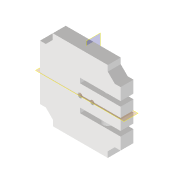
# Autodesk Inventor part: 20_Cube_Insert_2D_Galvo_Fiberlaunch_v3
Saved by Autodesk Inventor 2022 (Build 260153000, 153)
## iProperties
Created: 2019-07-01
Part Number: 20_Cube_Insert_2D_Galvo_Fiberlaunch_v3
Material: Generic
Document SubType Name: Modeling
Designer: diederichbenedict
Density: 1 g/cm^3
Appearance: Default
Author: diederichbenedict
Autodesk Inventor part; units mm, degrees
ref_plane "YZ Plane" through (0, 0, 0) normal (1, 0, 0) x (0, 1, 0)
ref_plane "XZ Plane" through (0, 0, 0) normal (0, 1, 0) x (-1, 0, 0)
ref_plane "Work Plane1" through (-56.3599, 0, 22) normal (0, 0, -1) x (-1, 0, 0)
sketch "Sketch1" plane through (-56.3599, 0, 22) normal (0, 0, -1) x (-1, 0, 0)
  line L0 (-4.0299, -0.3538) -> (-2.2322, 1.4439) construction
  arc A0 (-1.4439, 2.2322) -> (-2.2322, 1.4439) centre (-0.9299, 0.9299) ccw construction
  line L1 (-1.4439, 2.2322) -> (0.3538, 4.0299) construction
  line L2 (-37.8299, 42.8299) -> (-37.8299, 37.8299) construction
  line L3 (-37.8299, 37.8299) -> (-42.9208, 37.8299) construction
  line L4 (-37.8299, 42.2137) -> (-37.8299, 45.8299) construction
  line L5 (-37.8299, 45.8299) -> (-4.0299, 45.8299) construction
  line L6 (-4.0299, 45.8299) -> (-4.0299, 42.2137) construction
  line L7 (-4.0299, 4.0299) -> (0.3538, 4.0299) projected
  circle A1 centre (-20.9299, 20.9299) radius 17.5 projected
  line L8 (-20.9299, 58.9723) -> (17.1124, 20.9299) construction
  line L9 (17.1124, 20.9299) -> (-20.9299, -17.1124) construction
  line L10 (-20.9299, -17.1124) -> (-58.9723, 20.9299) construction
  line L11 (-58.9723, 20.9299) -> (-20.9299, 58.9723) construction
  line L12 (-20.9299, 58.9723) -> (-20.9299, -17.1124) construction
  line L13 (17.1124, 20.9299) -> (-58.9723, 20.9299) construction
  line L14 (-20.9299, 58.9723) -> (32.8701, 58.9723) construction
  line L15 (-43.4299, 43.4299) -> (1.5701, 43.4299) construction
  line L16 (1.5701, 43.4299) -> (1.5701, -1.5701) construction
  line L17 (1.5701, -1.5701) -> (-43.4299, -1.5701) construction
  line L18 (-43.4299, -1.5701) -> (-43.4299, 43.4299) construction
  line L19 (-43.4299, 43.4299) -> (1.5701, -1.5701) construction
  line L20 (1.5701, 43.4299) -> (-43.4299, -1.5701) construction
  line L21 (-43.4299, 5.3876) -> (-43.4299, 36.4723)
  line L22 (-43.4299, 36.4723) -> (-36.4723, 43.4299)
  line L23 (-36.4723, 43.4299) -> (-5.3876, 43.4299)
  line L24 (-5.3876, 43.4299) -> (1.5701, 36.4723)
  line L25 (1.5701, 36.4723) -> (1.5701, 5.3876)
  line L26 (1.5701, 5.3876) -> (-5.3876, -1.5701)
  line L27 (-5.3876, -1.5701) -> (-36.4723, -1.5701)
  line L28 (-36.4723, -1.5701) -> (-43.4299, 5.3876)
  line L29 (-4.0299, 42.2137) -> (-37.8299, 42.2137) projected
  line L30 (-4.0299, -0.3538) -> (-4.0299, 4.0299) projected
  circle A2 centre (-20.9299, 20.9299) radius 1.5
  line L31 (-10.9299, 10.9299) -> (-30.9299, 10.9299) construction
  line L32 (-30.9299, 10.9299) -> (-30.9299, 30.9299) construction
  line L33 (-30.9299, 30.9299) -> (-10.9299, 30.9299) construction
  line L34 (-10.9299, 30.9299) -> (-10.9299, 10.9299) construction
  line L35 (-10.9299, 10.9299) -> (-30.9299, 30.9299) construction
  line L36 (-30.9299, 10.9299) -> (-10.9299, 30.9299) construction
  circle A3 centre (-30.9299, 30.9299) radius 1.4
  circle A4 centre (-30.9299, 10.9299) radius 1.4
  circle A5 centre (-10.9299, 10.9299) radius 1.4
  line L37 (-45.8299, 37.8299) -> (-42.0723, 37.8299) construction
  line L38 (-42.1723, 37.7299) -> (-45.8299, 37.7299)
  line L39 (-45.8299, 37.7299) -> (-45.8299, 4.1299)
  line L40 (-45.8299, 4.1299) -> (-42.1723, 4.1299)
  line L41 (-42.1723, 4.1299) -> (-42.1723, 37.7299)
  line L42 (-45.8299, 4.0299) -> (-42.0723, 4.0299) construction
  line L43 (-45.8299, 37.8299) -> (-42.0723, 37.8299) projected
  line L44 (-37.7299, 45.8299) -> (-4.1299, 45.8299)
  line L45 (-4.1299, 45.8299) -> (-4.1299, 42.1723)
  line L46 (-4.1299, 42.1723) -> (-37.7299, 42.1723)
  line L47 (-37.7299, 42.1723) -> (-37.7299, 45.8299)
  line L48 (0.4701, 37.8299) -> (0.4701, 4.0299) construction
  line L49 (0.4701, 4.0299) -> (3.9701, 4.0299) construction
  line L50 (3.9701, 37.8299) -> (3.9701, 4.0299) construction
  line L51 (0.4701, 37.8299) -> (3.9701, 37.8299) construction
  line L52 (-45.8299, -3.9701) -> (-4.0299, -3.9701) construction
  line L53 (0.3124, 37.7299) -> (3.9701, 37.7299)
  line L54 (3.9701, 37.7299) -> (3.9701, 4.1299)
  line L55 (3.9701, 4.1299) -> (0.3124, 4.1299)
  line L56 (0.3124, 4.1299) -> (0.3124, 37.7299)
  line L57 (-4.1713, -0.3538) -> (-37.7299, -0.3538)
  line L58 (-37.7299, -0.3538) -> (-37.7299, -3.9701)
  line L59 (-37.7299, -3.9701) -> (-4.1713, -3.9701)
  line L60 (-4.1713, -3.9701) -> (-4.1713, -0.3538)
  point P0 (-37.8299, 4.0299)
  dimension "d18" = 53.8
  dimension "d19" = 45
  dimension "d20" = 53.8
  dimension "d21" = 45
  dimension "d22" = 45
  dimension "d30" = 20
  dimension "d31" = 20
  dimension "d32" = 2.8
  dimension "d33" = 2.8
  dimension "d34" = 2.8
  dimension "d35" = 3
  dimension "d36" = 0.1
  dimension "d37" = 0.1
  dimension "d38" = 0.1
  dimension "d39" = 0.1
  constraints: 86 end point, 21 point on line, 14 parallel, 8 perpendicular, 7 horizontal, 7 midpoint, 4 centre point, 4 coincident, 1 equal length
  measures "d18" distance of L8.start L8.end
  measures "d19" angle of L8 L14
  measures "d20" distance of L8.end L9.end
  measures "d21" distance of L16.end L17.end
  measures "d22" distance of L15.end L16.end
  measures "d30" distance of L32.end L33.end
  measures "d31" distance of L31.end L32.end
  measures "d32" diameter of A3
  measures "d33" diameter of A4
  measures "d34" diameter of A5
  measures "d35" diameter of A2
  measures "d36" distance between parallel lines of L38 L43
  measures "d37" distance between parallel lines of L40 L42
  measures "d38" distance between parallel lines of L45 L6
  measures "d39" distance between parallel lines of L4 L47
extrude "Extrusion1" add sketch "Sketch1" along normal blind 8 contours L30 L26 L57 L28 L41 L22 L46 L24 L56 L7 | L7 L26 L30 | L56 L24 L25 L26 | L26 L25 L24 L53 L54 L55 | L60 L59 L58 L57 L28 L27 L26 | L26 L27 L28 L57 | L46 L22 L29 L24 | L24 L29 L45 | L40 L39 L38 L22 L21 L28 | L28 L21 L22 L41 | L29 L22 L23 L24 | L24 L23 L22 L29 L47 L44 L45 | L47 L29 L22 | A1 | A2 | A3 | A4 | A5
sketch "Skizze4" plane through (-56.3599, 0, 14) normal (0, 0, -1) x (-1, 0, 0)
  line L0 (-37.7299, 42.1723) -> (-42.1723, 37.7299) projected
  line L1 (-42.1723, 37.7299) -> (-45.8299, 37.7299) projected
  line L2 (-45.8299, 37.7299) -> (-45.8299, 4.1299) construction
  line L3 (-45.8299, 4.1299) -> (-42.1723, 4.1299) projected
  line L4 (-42.1723, 4.1299) -> (-37.6885, -0.3538) projected
  line L5 (-37.6885, -0.3538) -> (-37.7299, -0.3538) projected
  line L6 (-37.7299, -0.3538) -> (-37.7299, -3.9701) projected
  line L7 (-37.7299, -3.9701) -> (-4.1713, -3.9701) construction
  line L8 (-4.1713, -3.9701) -> (-4.1713, -0.3538) projected
  line L9 (-4.1713, -0.3538) -> (0.3124, 4.1299) projected
  line L10 (0.3124, 4.1299) -> (3.9701, 4.1299) projected
  line L11 (3.9701, 4.1299) -> (3.9701, 37.7299) construction
  line L12 (3.9701, 37.7299) -> (0.3124, 37.7299) projected
  line L13 (0.3124, 37.7299) -> (-4.1299, 42.1723) projected
  line L14 (-4.1299, 42.1723) -> (-4.1299, 45.8299) projected
  line L15 (-4.1299, 45.8299) -> (-37.7299, 45.8299) construction
  line L16 (-37.7299, 45.8299) -> (-37.7299, 42.1723) projected
  line L17 (-37.9299, 46.0299) -> (-3.9299, 46.0299) construction
  line L18 (-3.9299, 46.0299) -> (-3.9299, 42.2551)
  line L19 (-3.9299, 42.2551) -> (0.3953, 37.9299)
  line L20 (0.3953, 37.9299) -> (4.1701, 37.9299)
  line L21 (4.1701, 37.9299) -> (4.1701, 3.9299) construction
  line L22 (4.1701, 3.9299) -> (0.3953, 3.9299)
  line L23 (0.3953, 3.9299) -> (-3.9713, -0.4367)
  line L24 (-3.9713, -0.4367) -> (-3.9713, -4.1701)
  line L25 (-3.9713, -4.1701) -> (-37.9299, -4.1701) construction
  line L26 (-37.9299, -4.1701) -> (-37.9299, -0.3953)
  line L27 (-37.9299, -0.3953) -> (-42.2551, 3.9299)
  line L28 (-42.2551, 3.9299) -> (-46.0299, 3.9299)
  line L29 (-46.0299, 3.9299) -> (-46.0299, 37.9299) construction
  line L30 (-46.0299, 37.9299) -> (-42.2551, 37.9299)
  line L31 (-42.2551, 37.9299) -> (-37.9299, 42.2551)
  line L32 (-37.9299, 42.2551) -> (-37.9299, 46.0299)
  line L33 (-45.8299, 37.7299) -> (-45.8299, 37.9299)
  line L34 (-4.1299, 45.8299) -> (-37.7299, 45.8299) projected
  line L35 (-37.7299, 45.8299) -> (-37.9299, 45.8299)
  line L36 (-4.1299, 45.8299) -> (-3.9299, 45.8299)
  line L37 (3.9701, 37.7299) -> (3.9701, 37.9299)
  line L38 (3.9701, 4.1299) -> (3.9701, 37.7299) projected
  line L39 (3.9701, 4.1299) -> (3.9701, 3.9299)
  line L40 (-4.1713, -3.9701) -> (-3.9713, -3.9701)
  line L41 (-37.7299, -3.9701) -> (-37.9299, -3.9701)
  line L42 (-45.8299, 4.1299) -> (-45.8299, 3.9299)
  point P0 (-56.3599, 0)
  dimension "d40" = 0.2
  constraints: 48 end point, 12 point on line, 4 perpendicular, 15 other
  measures "d40" distance between parallel lines of L15 L17
extrude "IM_offset" add sketch "Skizze4" against normal up to surface (8 mm away)
ref_plane "Arbeitsebene5" through (-35.4299, 3.9299, 22) normal (-1, 0, 0) x (0, 0, 1)
ref_plane "Arbeitsebene6" through (-18.4299, 20.9299, 22) normal (0, 1, 0) x (-1, 0, 0)
sketch "Skizze31" plane through (-56.3599, 0, 22) normal (0, 0, 1) x (1, 0, 0)
  line L0 (25.9049, 44.8899) -> (15.7949, 44.8899) projected
  spline S0 degree 3 poles (21.2744, 21.9194) (21.3357, 21.9462) (21.3936, 21.9718) (21.5033, 22.0154) (21.5491, 22.0289) (21.5827, 22.0289) (21.5892, 22.0276) (21.5935, 22.0247) knots 0.300335 0.300335 0.300335 0.300335 0.323424 0.323424 0.35266 0.35266 0.362351 0.362351 0.362351 0.362351 projected
  line L1 (21.2744, 21.9194) -> (21.2744, 26.3899) projected
  line L2 (20.4254, 21.9194) -> (20.4254, 26.3899) projected
  line L3 (21.9714, 15.3899) -> (21.1087, 15.3899) projected
  line L4 (20.5911, 15.3899) -> (19.7285, 15.3899) projected
  line L5 (20.5999, 15.3899) -> (21.0999, 15.3899) projected
  line L6 (28.5999, 22.8289) -> (28.5999, 24.3299) projected
  line L7 (28.5999, 24.3299) -> (28.0999, 24.3299) projected
  line L8 (28.0999, 24.3299) -> (28.0999, 22.8289) projected
  line L9 (28.0999, 22.8289) -> (27.7114, 24.2788) projected
  line L10 (27.7114, 24.2788) -> (27.2285, 24.1494) projected
  line L11 (27.2285, 24.1494) -> (28.0911, 20.9299) projected
  line L12 (28.0911, 20.9299) -> (27.2285, 17.7105) projected
  line L13 (27.2285, 17.7105) -> (27.7114, 17.5811) projected
  line L14 (27.7114, 17.5811) -> (28.0999, 19.031) projected
  line L15 (28.0999, 19.031) -> (28.0999, 17.5299) projected
  line L16 (28.0999, 17.5299) -> (28.5999, 17.5299) projected
  line L17 (28.5999, 17.5299) -> (28.5999, 19.031) projected
  line L18 (28.5999, 19.031) -> (28.9884, 17.5811) projected
  line L19 (28.9884, 17.5811) -> (29.4714, 17.7105) projected
  line L20 (29.4714, 17.7105) -> (28.6087, 20.9299) projected
  line L21 (28.6087, 20.9299) -> (29.4714, 24.1494) projected
  line L22 (29.4714, 24.1494) -> (28.9884, 24.2788) projected
  line L23 (28.9884, 24.2788) -> (28.5999, 22.8289) projected
  circle A0 centre (28.3499, 20.9299) radius 1.35
  line L24 (3.9713, -3.9701) -> (37.9299, -3.9701) projected
  line L25 (37.9299, -3.9701) -> (37.9299, -0.3953) projected
  line L26 (37.9299, -0.3953) -> (42.2551, 3.9299) projected
  line L27 (42.2551, 3.9299) -> (45.8299, 3.9299) projected
  line L28 (45.8299, 3.9299) -> (45.8299, 37.9299) projected
  line L29 (45.8299, 37.9299) -> (42.2551, 37.9299) projected
  line L30 (42.2551, 37.9299) -> (37.9299, 42.2551) projected
  line L31 (37.9299, 42.2551) -> (37.9299, 45.8299) projected
  line L32 (37.9299, 45.8299) -> (3.9299, 45.8299) projected
  line L33 (3.9299, 45.8299) -> (3.9299, 42.2551) projected
  line L34 (3.9299, 42.2551) -> (-0.3953, 37.9299) projected
  line L35 (-0.3953, 37.9299) -> (-3.9701, 37.9299) projected
  line L36 (-3.9701, 37.9299) -> (-3.9701, 3.9299) projected
  line L37 (-3.9701, 3.9299) -> (-0.3953, 3.9299) projected
  line L38 (-0.3953, 3.9299) -> (3.9713, -0.4367) projected
  line L39 (3.9713, -0.4367) -> (3.9713, -3.9701) projected
  line L40 (45.8299, 37.9299) -> (45.8299, 3.9299) projected
  line L41 (20.8299, 20.4299) -> (45.8299, 20.4299)
  line L42 (45.8299, 20.4299) -> (45.8299, 21.4299)
  line L43 (45.8299, 21.4299) -> (20.8299, 21.4299)
  line L44 (20.8299, 21.4299) -> (20.8299, 20.4299)
  line L45 (20.8299, 20.4299) -> (45.8299, 21.4299) construction
  line L46 (45.8299, 20.4299) -> (20.8299, 21.4299) construction
  line L47 (45.8299, 30.4299) -> (20.8299, 30.4299)
  line L48 (20.8299, 30.4299) -> (20.8299, 27.4299)
  line L49 (20.8299, 27.4299) -> (45.8299, 27.4299)
  line L50 (45.8299, 27.4299) -> (45.8299, 30.4299)
  line L51 (45.8299, 14.4299) -> (20.8299, 14.4299)
  line L52 (20.8299, 14.4299) -> (20.8299, 11.4299)
  line L53 (20.8299, 11.4299) -> (45.8299, 11.4299)
  line L54 (45.8299, 11.4299) -> (45.8299, 14.4299)
  circle A1 centre (20.8299, 20.9299) radius 1.5
  point P0 (56.3599, 0)
  point P1 (33.3299, 20.9299)
  point P2 (45.8299, 11.4299)
  point P3 (27.0959, 20.4299)
  point P4 (29.6039, 20.4299)
  point P5 (29.6039, 21.4299)
  point P6 (27.0959, 21.4299)
  point P7 (22.2441, 21.4299)
  point P8 (22.2441, 20.4299)
  point P9 (45.8299, 27.4299)
  dimension "d181" = 2.7
  dimension "d182" = 1
  dimension "d183" = 3
  dimension "d184" = 3
  dimension "d185" = 25
  dimension "d186" = 0
  dimension "d187" = 3
  dimension "d197" = 6
  dimension "d198" = 6
  constraints: 28 end point, 6 parallel, 4 point on line, 3 horizontal, 3 midpoint, 3 perpendicular, 2 centre point
  measures "d181" diameter of A0
  measures "d182" distance of L42.end L41.end
  measures "d183" distance of L48.end L47.end
  measures "d184" distance of L52.end L51.end
  measures "d185" distance between parallel lines of L48 L40
  measures "d186" distance between parallel lines of L52 L44
  measures "d187" diameter of A1
  measures "d197" distance between parallel lines of L43 L49
  measures "d198" distance between parallel lines of L51 L41
extrude "Extrusion26" cut sketch "Skizze31" against normal blind 10 contours A0 L43 L21 | L21 L43 L11 A0 | L43 A0 L41 L20 L21 | L21 L20 L41 L12 L11 L43 | L43 L28 L41 A0 | L11 L43 A0 | L11 L12 L41 A0 L43 | A0 L41 A1 L43 | L41 A0 L20 | L20 A0 L12 L41 | L49 L48 L47 L28 | L41 L12 A0 | A1 L41 L44 L43 | L43 L44 L41 A1 | L28 L53 L52 L51
sketch "Skizze32" plane through (-35.5299, -3.9701, 22) normal (0, -1, 0) x (1, 0, 0)
  line L0 (8.774, 0) -> (8.774, -8) projected
  line L1 (6.266, 0) -> (6.266, -8) projected
  line L2 (-16.8586, 0) -> (17.1, 0) projected
  line L3 (-16.8586, -8) -> (-16.8586, 0) projected
  line L4 (-16.8586, -8) -> (17.1, -8) projected
  line L5 (17.1, -8) -> (17.1, 0) projected
  circle A0 centre (13.0607, -4) radius 0.7419
  point P0 (35.5299, -22)
  constraints: 1 centre point
hole "Bohrung2" at (-22.4692, -3.9701, 18) direction (0, 1, 0) diameter 2.8 depth 35 tip angle 118 counterbore diameter 6.5 counterbore depth 16
body "Solid1"
